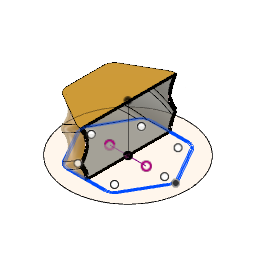
Short Hexagon Twist R50 H50 O10 I10 C65 (Autodesk Fusion 360 design; units mm, degrees)
Autodesk Fusion 360 part; units mm, degrees
sketch "Base Profile" plane through (0, 0, 0) normal (0, 0, 1) x (1, 0, 0)
  line L0 (47.1132, 5) -> (27.8868, 38.3013)
  line L1 (19.2265, 43.3013) -> (-19.2265, 43.3013)
  line L2 (-27.8868, 38.3013) -> (-47.1132, 5)
  line L3 (-47.1132, -5) -> (-27.8868, -38.3013)
  line L4 (-19.2265, -43.3013) -> (19.2265, -43.3013)
  line L5 (27.8868, -38.3013) -> (47.1132, -5)
  arc A0 (-19.2265, 43.3013) -> (-27.8868, 38.3013) centre (-19.2265, 33.3013) ccw
  arc A1 (27.8868, 38.3013) -> (19.2265, 43.3013) centre (19.2265, 33.3013) ccw
  arc A2 (-47.1132, 5) -> (-47.1132, -5) centre (-38.453, 0) ccw
  arc A3 (-27.8868, -38.3013) -> (-19.2265, -43.3013) centre (-19.2265, -33.3013) ccw
  arc A4 (19.2265, -43.3013) -> (27.8868, -38.3013) centre (19.2265, -33.3013) ccw
  arc A5 (47.1132, -5) -> (47.1132, 5) centre (38.453, 0) ccw
  line L6 (-19.2265, -43.9513) -> (19.2265, -43.9513)
  arc A6 (19.2265, -43.9513) -> (28.4497, -38.6263) centre (19.2265, -33.3013) ccw
  line L7 (28.4497, -38.6263) -> (47.6762, -5.325)
  arc A7 (47.6762, -5.325) -> (47.6762, 5.325) centre (38.453, 0) ccw
  line L8 (47.6762, 5.325) -> (28.4497, 38.6263)
  arc A8 (28.4497, 38.6263) -> (19.2265, 43.9513) centre (19.2265, 33.3013) ccw
  line L9 (19.2265, 43.9513) -> (-19.2265, 43.9513)
  arc A9 (-19.2265, 43.9513) -> (-28.4497, 38.6263) centre (-19.2265, 33.3013) ccw
  line L10 (-28.4497, 38.6263) -> (-47.6762, 5.325)
  arc A10 (-47.6762, 5.325) -> (-47.6762, -5.325) centre (-38.453, 0) ccw
  line L11 (-47.6762, -5.325) -> (-28.4497, -38.6263)
  arc A11 (-28.4497, -38.6263) -> (-19.2265, -43.9513) centre (-19.2265, -33.3013) ccw
  line L12 (27.0207, -37.8013) -> (46.2472, -4.5)
  arc A12 (46.2472, -4.5) -> (46.2472, 4.5) centre (38.453, 0) ccw
  line L13 (46.2472, 4.5) -> (27.0207, 37.8013)
  arc A13 (27.0207, 37.8013) -> (19.2265, 42.3013) centre (19.2265, 33.3013) ccw
  line L14 (19.2265, 42.3013) -> (-19.2265, 42.3013)
  arc A14 (-19.2265, 42.3013) -> (-27.0207, 37.8013) centre (-19.2265, 33.3013) ccw
  line L15 (-27.0207, 37.8013) -> (-46.2472, 4.5)
  arc A15 (-46.2472, 4.5) -> (-46.2472, -4.5) centre (-38.453, 0) ccw
  line L16 (-46.2472, -4.5) -> (-27.0207, -37.8013)
  arc A16 (-27.0207, -37.8013) -> (-19.2265, -42.3013) centre (-19.2265, -33.3013) ccw
  line L17 (-19.2265, -42.3013) -> (19.2265, -42.3013)
  arc A17 (19.2265, -42.3013) -> (27.0207, -37.8013) centre (19.2265, -33.3013) ccw
  line L18 (29.3157, -39.1263) -> (48.5422, -5.825)
  arc A18 (48.5422, -5.825) -> (48.5422, 5.825) centre (38.453, 0) ccw
  line L19 (48.5422, 5.825) -> (29.3157, 39.1263)
  arc A19 (29.3157, 39.1263) -> (19.2265, 44.9513) centre (19.2265, 33.3013) ccw
  line L20 (19.2265, 44.9513) -> (-19.2265, 44.9513)
  arc A20 (-19.2265, 44.9513) -> (-29.3157, 39.1263) centre (-19.2265, 33.3013) ccw
  line L21 (-29.3157, 39.1263) -> (-48.5422, 5.825)
  arc A21 (-48.5422, 5.825) -> (-48.5422, -5.825) centre (-38.453, 0) ccw
  line L22 (-48.5422, -5.825) -> (-29.3157, -39.1263)
  arc A22 (-29.3157, -39.1263) -> (-19.2265, -44.9513) centre (-19.2265, -33.3013) ccw
  line L23 (-19.2265, -44.9513) -> (19.2265, -44.9513)
  arc A23 (19.2265, -44.9513) -> (29.3157, -39.1263) centre (19.2265, -33.3013) ccw
  circle A24 centre (0, 0) radius 62.5
  dimension "d1" = 50
  dimension "d2" = 0.65
  dimension "d3" = 1
  dimension "d4" = 1.65
  dimension "d12" = 10
  dimension "d34" = 125
  measures "d2" distance of L4
  measures "d3" distance of L5
  measures "d4" distance of L5
  measures "d12" radius of A0
  measures "d34" diameter of A24
sketch "Vertical Path" plane through (0, 0, 0) normal (0, 1, 0) x (1, 0, 0)
  line L0 (19.2265, 0) -> (-19.2265, 0)
  line L1 (0, 0) -> (0, -50)
  dimension "d8" = 50
sweep "Sweep1" add twist angle 90 profiles "Base Profile" path "Vertical Path" along L1 section 1 contours L0 L1 L2 L3 L4 L5 A0 A1 A2 A3 A4 A5 makes body 1
sweep "Sweep2" add twist angle 90 profiles "Base Profile" path "Vertical Path" along L1 section 1 contours L18 A18 L19 A19 L20 A20 L21 A21 L22 A22 L23 A23 separate body makes body 2
ref_plane "WorkPlane1" through (0, 0, 50) normal (0, 0, 1) x (1, 0, 0)
sweep "Sweep3" add twist angle 90 profiles "Base Profile" path "Vertical Path" along L1 section 1 contours L12 A12 L13 A13 L14 A14 L15 A15 L16 A16 L17 A17 separate body makes body 3
extrude "Extrude2" cut sketch "Base Profile" along normal blind 50 from surface at 1 contours L0 L1 L2 L3 L4 L5 A0 A1 A2 A3 A4 A5 | L6 A6 L7 A7 L8 A8 L9 A9 L10 A10 L11 A11 | L12 A12 L13 A13 L14 A14 L15 A15 L16 A16 L17 A17 | L18 A18 L19 A19 L20 A20 L21 A21 L22 A22 L23 A23 | A24 bodies 3
sweep "Sweep4" add twist angle 90 profiles "Base Profile" path "Vertical Path" along L1 section 1 contours L0 L1 L2 L3 L4 L5 A0 A1 A2 A3 A4 A5 | L6 A6 L7 A7 L8 A8 L9 A9 L10 A10 L11 A11 | L12 A12 L13 A13 L14 A14 L15 A15 L16 A16 L17 A17 | L18 A18 L19 A19 L20 A20 L21 A21 L22 A22 L23 A23 separate body makes body 4
sketch "Sketch4" plane through (0, 0, 50) normal (0, 0, 1) x (-1, 0, 0)
  arc A0 (-44.9513, -19.2265) -> (-39.1263, -29.3157) centre (-33.3013, -19.2265) ccw
  line L0 (-39.1263, -29.3157) -> (-5.825, -48.5422)
  arc A1 (-5.825, -48.5422) -> (5.825, -48.5422) centre (0, -38.453) ccw
  line L1 (5.825, -48.5422) -> (39.1263, -29.3157)
  arc A2 (39.1263, -29.3157) -> (44.9513, -19.2265) centre (33.3013, -19.2265) ccw
  line L2 (44.9513, -19.2265) -> (44.9513, 19.2265)
  arc A3 (44.9513, 19.2265) -> (39.1263, 29.3157) centre (33.3013, 19.2265) ccw
  line L3 (39.1263, 29.3157) -> (5.825, 48.5422)
  arc A4 (5.825, 48.5422) -> (-5.825, 48.5422) centre (0, 38.453) ccw
  line L4 (-5.825, 48.5422) -> (-39.1263, 29.3157)
  arc A5 (-39.1263, 29.3157) -> (-44.9513, 19.2265) centre (-33.3013, 19.2265) ccw
  line L5 (-44.9513, 19.2265) -> (-44.9513, -19.2265)
  circle A6 centre (0, 0) radius 53.0456
extrude "Extrude6" cut sketch "Sketch4" against normal blind 1 contours A0 L0 A1 L1 A2 L2 A3 L3 A4 L4 A5 L5 | A6 keep common part bodies 4
extrude "Extrude7" cut sketch "Sketch4" against normal blind 1.65 contours A0 L0 A1 L1 A2 L2 A3 L3 A4 L4 A5 L5 | A6 bodies 1
combine "Combine1" operation add target body 3 tool bodies 1
combine "Combine2" operation add target body 4 tool bodies 2
sketch "Sketch5" plane through (0, 0, 0) normal (1, 0, 0) x (0, 1, 0)
  line L0 (-60, 50) -> (83.8935, 50)
  line L1 (83.8935, 50) -> (83.8935, -7.0403)
  line L2 (83.8935, -7.0403) -> (-60, -7.0403)
  line L3 (-60, -7.0403) -> (-60, 50)
ref_plane "WorkPlane2" through (0, 11.9468, 21.4799) normal (1, 0, 0) x (0, 1, 0)
equation "d1 = Radius"
equation "d2 = Clearance"
equation "d3 = Thickness"
equation "d4 = Clearance + Thickness"
equation "Clearance = 0.65 mm"
equation "Height = 50 mm"
equation "Radius = 50 mm"
equation "d8 = Height"
equation "Thickness = 1 mm"
equation "Twist = 90 deg"
equation "Fillet = 10 mm"
equation "d12 = Fillet"
equation "d17 = Twist"
equation "d23 = Twist"
equation "d27 = Height"
equation "d32 = Twist"
equation "d34 = Radius * 2.5"
equation "d35 = Thickness"
equation "d36 = Height"
equation "d45 = Twist"
equation "d52 = -Thickness"
equation "d54 = -Thickness - Clearance"
named bodies: "Inner Shell", "Outer Shell", "Inner", "Outer"
